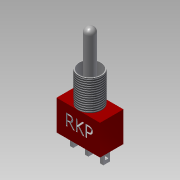
# Autodesk Inventor part: Saklar
Saved by Autodesk Inventor 2015 SP1 (Build 190203100, 203)
## iProperties
Created: 2015-02-14
Part Number: Saklar
Material: Generic
Document SubType Name: Modeling
Designer: Rafi Kurnia Putra
Density: 1 g/cm^3
Appearance: Steel
Author: Rafi Kurnia Putra
Autodesk Inventor part; units mm, degrees
ref_plane "YZ Plane" through (0, 0, 0) normal (1, 0, 0) x (0, 1, 0)
ref_plane "XZ Plane" through (0, 0, 0) normal (0, 1, 0) x (-1, 0, 0)
ref_plane "XY Plane" through (0, 0, 0) normal (0, 0, 1) x (1, 0, 0)
sketch "Sketch1" plane through (0, 0, 0) normal (0, 1, 0) x (-1, 0, 0)
  line L0 (6.5, -3.5) -> (-6.5, -3.5)
  line L1 (-6.5, -3.5) -> (-6.5, 3.5)
  line L2 (-6.5, 3.5) -> (6.5, 3.5)
  line L3 (6.5, 3.5) -> (6.5, -3.5)
  line L4 (6.5, -3.5) -> (-6.5, 3.5) construction
  line L5 (-6.5, -3.5) -> (6.5, 3.5) construction
  point P0 (0, 0)
  dimension "d0" = 13
  dimension "d1" = 7
  constraints: 12 end point, 2 midpoint, 2 parallel, 1 horizontal, 1 perpendicular
  measures "d0" distance of L1.end L2.end
  measures "d1" distance of L0.end L1.end
extrude "Extrusion1" add sketch "Sketch1" along normal blind 9
sketch "Sketch2" plane through (0, 9, 0) normal (0, 1, 0) x (1, 0, 0)
  circle A0 centre (0, 0) radius 3.5
  dimension "d4" = 7
  constraints: 1 centre point, 1 coincident
  measures "d4" diameter of A0
extrude "Extrusion2" add sketch "Sketch2" along normal blind 9
thread "Thread1" size "M3.5x0.6" class "6g" standard "ANSI Metric M Profile" full length
sketch "Sketch3" plane through (0, 0, 0) normal (0, -1, 0) x (1, 0, 0)
  line L0 (0.5, -1) -> (-0.5, -1)
  line L1 (-0.5, -1) -> (-0.5, 1)
  line L2 (-0.5, 1) -> (0.5, 1)
  line L3 (0.5, 1) -> (0.5, -1)
  line L4 (0.5, -1) -> (-0.5, 1) construction
  line L5 (-0.5, -1) -> (0.5, 1) construction
  line L6 (-6.5, -3.5) -> (6.5, -3.5) projected
  line L7 (5, -1) -> (4, -1)
  line L8 (4, -1) -> (4, 1)
  line L9 (4, 1) -> (5, 1)
  line L10 (5, 1) -> (5, -1)
  line L11 (5, -1) -> (4, 1) construction
  line L12 (4, -1) -> (5, 1) construction
  line L13 (-4, -1) -> (-5, -1)
  line L14 (-5, -1) -> (-5, 1)
  line L15 (-5, 1) -> (-4, 1)
  line L16 (-4, 1) -> (-4, -1)
  line L17 (-4, -1) -> (-5, 1) construction
  line L18 (-5, -1) -> (-4, 1) construction
  line L19 (0.5, -1) -> (-0.5, -1)
  line L20 (-0.5, -1) -> (-0.5, 1)
  line L21 (-0.5, 1) -> (0.5, 1)
  line L22 (0.5, 1) -> (0.5, -1)
  line L23 (0.5, -1) -> (-0.5, 1) construction
  line L24 (-0.5, -1) -> (0.5, 1) construction
  point P0 (0, 0)
  dimension "d9" = 1
  dimension "d10" = 2
  dimension "d13" = 4.5
  dimension "d16" = 4.5
  constraints: 48 end point, 3 horizontal, 2 midpoint, 2 parallel, 1 perpendicular, 30 other
  measures "d9" distance of L1.end L2.end
  measures "d10" distance of L0.end L1.end
  measures "d13" distance of L0.start L7.start
  measures "d16" distance of L0.start L13.start
extrude "Extrusion3" add sketch "Sketch3" along normal blind 4
sketch "Sketch4" plane through (5, 0, 1) normal (1, 0, 0) x (0, 0, -1)
  line L0 (0, 0) -> (2, 0) projected
  line L1 (0, 0) -> (0, -4) projected
  line L2 (2, -4) -> (0, -4) projected
  line L3 (2, 0) -> (2, -4) projected
  line L4 (0.75, -3) -> (1.25, -3)
  line L5 (1.5, -2.75) -> (1.5, -1.25)
  line L6 (1.25, -1) -> (0.75, -1)
  line L7 (0.5, -1.25) -> (0.5, -2.75)
  line L8 (0.5, -3) -> (1.5, -1) construction
  line L9 (1.5, -3) -> (0.5, -1) construction
  arc A0 (0.75, -1) -> (0.5, -1.25) centre (0.75, -1.25) ccw
  arc A1 (1.5, -1.25) -> (1.25, -1) centre (1.25, -1.25) ccw
  arc A2 (1.25, -3) -> (1.5, -2.75) centre (1.25, -2.75) ccw
  arc A3 (0.5, -2.75) -> (0.75, -3) centre (0.75, -2.75) ccw
  point P0 (1, 0)
  point P1 (1, -2)
  dimension "d21" = 1
  dimension "d22" = 2
  dimension "d23" = 0.25
  constraints: 12 end point, 8 point on circle, 8 point on line, 8 tangent, 4 centre point, 3 equal radius, 2 midpoint, 2 parallel, 1 horizontal, 1 perpendicular
  measures "d21" distance of L9.end L8.end
  measures "d22" distance of L8.end L9.start
  measures "d23" radius of A0
extrude "Extrusion4" cut sketch "Sketch4" against normal through all contours A3 L7 A0 L6 A1 L5 A2 L4
shell "Shell1" thickness 0.3 removed faces 1 at (-0.4137, 18, -0.4564)
sketch "Sketch5" plane through (0, 9, 0) normal (0, 1, 0) x (1, 0, 0)
  circle A0 centre (0, 0) radius 1.5
  dimension "d27" = 3
  constraints: 1 centre point, 1 coincident
  measures "d27" diameter of A0
extrude "Extrusion5" add sketch "Sketch5" along normal blind 20
fillet "Fillet1" radius 1.5 1 edges at (-1.5, 29, 0)
sketch "Sketch6" plane through (6.5, 0, -3.5) normal (0, 0, -1) x (-1, 0, 0)
  line L0 (2.4376, 6.6133) -> (10.9096, 6.6133) construction
  line L1 (10.9096, 6.6133) -> (10.9096, 3.1133) construction
  line L2 (10.9096, 3.1133) -> (2.4376, 3.1133) construction
  line L3 (2.4376, 3.1133) -> (2.4376, 6.6133) construction
  line L4 (5.5008, 3.1133) -> (4.8966, 3.1133)
  line L5 (4.8966, 3.1133) -> (3.7905, 4.5059)
  line L6 (3.7905, 4.5059) -> (3.2573, 4.5059)
  line L7 (3.2573, 4.5059) -> (3.2573, 3.1133)
  line L8 (3.2573, 3.1133) -> (2.7921, 3.1133)
  line L9 (2.7921, 3.1133) -> (2.7921, 6.6133)
  line L10 (2.7921, 6.6133) -> (3.6941, 6.6133)
  spline S0 degree 2 poles (3.6941, 6.6133) (3.9947, 6.6133) (4.4003, 6.548) (4.5847, 6.4289) knots 0 0 0 1 2 2 2
  spline S1 degree 2 poles (4.5847, 6.4289) (4.769, 6.3098) (4.9817, 5.9382) (4.9817, 5.6631) knots 0 0 0 1 2 2 2
  spline S2 degree 2 poles (4.9817, 5.6631) (4.9817, 5.2802) (4.5903, 4.7611) (4.2556, 4.6363) knots 0 0 0 1 2 2 2
  line L11 (4.2556, 4.6363) -> (5.5008, 3.1133)
  spline S3 degree 2 poles (4.4967, 5.6262) (4.4967, 5.7794) (4.389, 6.0148) (4.2755, 6.0914) knots 0 0 0 1 2 2 2
  spline S4 degree 2 poles (4.2755, 6.0914) (4.1762, 6.1566) (3.9125, 6.2105) (3.7196, 6.2105) knots 0 0 0 1 2 2 2
  line L12 (3.7196, 6.2105) -> (3.2573, 6.2105)
  line L13 (3.2573, 6.2105) -> (3.2573, 4.8945)
  line L14 (3.2573, 4.8945) -> (3.6657, 4.8945)
  spline S5 degree 2 poles (3.6657, 4.8945) (3.8671, 4.8945) (4.1876, 4.9654) (4.2982, 5.076) knots 0 0 0 1 2 2 2
  spline S6 degree 2 poles (4.2982, 5.076) (4.4003, 5.1724) (4.4967, 5.4447) (4.4967, 5.6262) knots 0 0 0 1 2 2 2
  line L15 (8.3314, 3.1133) -> (7.7273, 3.1133)
  line L16 (7.7273, 3.1133) -> (6.4481, 4.7413)
  line L17 (6.4481, 4.7413) -> (6.2439, 4.5116)
  line L18 (6.2439, 4.5116) -> (6.2439, 3.1133)
  line L19 (6.2439, 3.1133) -> (5.7787, 3.1133)
  line L20 (5.7787, 3.1133) -> (5.7787, 6.6133)
  line L21 (5.7787, 6.6133) -> (6.2439, 6.6133)
  line L22 (6.2439, 6.6133) -> (6.2439, 5.0051)
  line L23 (6.2439, 5.0051) -> (7.6791, 6.6133)
  line L24 (7.6791, 6.6133) -> (8.2463, 6.6133)
  line L25 (8.2463, 6.6133) -> (6.797, 5.0504)
  line L26 (6.797, 5.0504) -> (8.3314, 3.1133)
  spline S7 degree 2 poles (10.8217, 5.5581) (10.8217, 5.3312) (10.66, 4.9228) (10.5154, 4.781) knots 0 0 0 1 2 2 2
  spline S8 degree 2 poles (10.5154, 4.781) (10.3338, 4.6023) (9.8432, 4.418) (9.4688, 4.418) knots 0 0 0 1 2 2 2
  line L27 (9.4688, 4.418) -> (9.0745, 4.418)
  line L28 (9.0745, 4.418) -> (9.0745, 3.1133)
  line L29 (9.0745, 3.1133) -> (8.6094, 3.1133)
  line L30 (8.6094, 3.1133) -> (8.6094, 6.6133)
  line L31 (8.6094, 6.6133) -> (9.4886, 6.6133)
  spline S9 degree 2 poles (9.4886, 6.6133) (9.8006, 6.6133) (10.2374, 6.5111) (10.4048, 6.3949) knots 0 0 0 1 2 2 2
  spline S10 degree 2 poles (10.4048, 6.3949) (10.6005, 6.2616) (10.8217, 5.8503) (10.8217, 5.5581) knots 0 0 0 1 2 2 2
  spline S11 degree 2 poles (10.3367, 5.544) (10.3367, 5.7255) (10.2119, 5.9921) (10.0842, 6.0772) knots 0 0 0 1 2 2 2
  spline S12 degree 2 poles (10.0842, 6.0772) (9.9736, 6.1509) (9.6787, 6.2105) (9.4603, 6.2105) knots 0 0 0 1 2 2 2
  line L32 (9.4603, 6.2105) -> (9.0745, 6.2105)
  line L33 (9.0745, 6.2105) -> (9.0745, 4.815)
  line L34 (9.0745, 4.815) -> (9.3922, 4.815)
  spline S13 degree 2 poles (9.3922, 4.815) (9.6758, 4.815) (10.0247, 4.9058) (10.1381, 5.0249) knots 0 0 0 1 2 2 2
  spline S14 degree 2 poles (10.1381, 5.0249) (10.2431, 5.1299) (10.3367, 5.3766) (10.3367, 5.544) knots 0 0 0 1 2 2 2
  point P0 (6.5, 0)
  constraints: 2 other
extrude "Extrusion6" cut sketch "Sketch6" against normal through all
body "Solid1"
